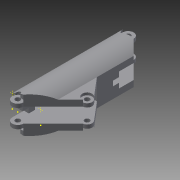
# Autodesk Inventor part: Finger_Lower_main_1
Saved by Autodesk Inventor 2015 (Build 190159000, 159)
## iProperties
Created: 2016-07-06
Part Number: Finger_Lower_main_1
Material: Generic
Document SubType Name: Modeling
Designer: Neelotpal Nag
Density: 1 g/cm^3
Appearance: Default
Author: Neelotpal Nag
Autodesk Inventor part; units mm, degrees
ref_plane "YZ Plane" through (0, 0, 0) normal (1, 0, 0) x (0, 1, 0)
ref_plane "XZ Plane" through (0, 0, 0) normal (0, 1, 0) x (-1, 0, 0)
sketch "Sketch1" plane through (0, 0, 0) normal (0, 0, 1) x (1, 0, 0)
  line L0 (0, 0) -> (0, 45)
  line L1 (0, 0) -> (14.1421, 14.1421)
  line L2 (0, 0) -> (20, 0) construction
  line L3 (14.1421, 14.1421) -> (0, 14.1421)
  circle A0 centre (0, 0) radius 1
  circle A1 centre (14.1421, 14.1421) radius 1
  circle A2 centre (0, 45) radius 1
  circle A3 centre (0, 0) radius 2.25
  circle A4 centre (0, 45) radius 2.25
  dimension "d0" = 45
  dimension "d1" = 20
  dimension "d2" = 45
  dimension "d3" = 2
  dimension "d4" = 2
  dimension "d5" = 2
  dimension "d6" = 4.5
  dimension "d10" = 4.5
  constraints: 8 coincident, 8 end point, 5 centre point, 1 equal length, 1 horizontal, 1 perpendicular, 1 point on line, 1 vertical
  measures "d0" distance of L0.start L0.end
  measures "d1" distance of L1.start L1.end
  measures "d2" angle of L2 L1
  measures "d3" diameter of A0
  measures "d4" diameter of A1
  measures "d5" diameter of A2
  measures "d6" diameter of A3
  measures "d10" diameter of A4
ref_plane "Work Plane1" through (0, 0, 3) normal (0, 0, 1) x (1, 0, 0)
sketch "Sketch2" plane through (0, 0, 3) normal (0, 0, 1) x (1, 0, 0)
  circle A0 centre (0, 0) radius 1 projected
  circle A1 centre (0, 0) radius 2.25 projected
  circle A2 centre (14.1421, 14.1421) radius 1 projected
  circle A3 centre (0, 45) radius 1 projected
  circle A4 centre (0, 45) radius 2.25 projected
  line L0 (0, 0) -> (0, 45) projected
extrude "Extrusion1" add sketch "Sketch2" along normal blind 1.5 contours A1
sketch "Sketch3" plane through (0, 0, 3) normal (0, 0, 1) x (1, 0, 0)
  point P0 (0, 0)
extrude "Extrusion2" add sketch "Sketch2" along normal blind 1.5 contours A4
sketch "Sketch4" plane through (0, 0, 3) normal (0, 0, 1) x (1, 0, 0)
  circle A0 centre (0, 0) radius 2.25 projected
  line L0 (-2.25, 0) -> (-2.25, 45)
  circle A1 centre (0, 45) radius 2.25 projected
  line L1 (2.25, 45) -> (9.3211, 37.9289)
  line L2 (2.25, 45) -> (12.25, 45) construction
  line L3 (9.3211, 37.9289) -> (9.3211, 22.9289)
  dimension "d13" = 10
  dimension "d14" = 45
  dimension "d15" = 15
  constraints: 8 end point, 2 point on circle, 1 equal length, 1 horizontal, 1 horizontal alignment, 1 parallel, 1 tangent, 1 vertical, 1 other
  measures "d13" distance of L1.start L1.end
  measures "d14" angle of L1 L2
  measures "d15" distance of L1.end L3.end
sketch "Sketch5" plane through (0, 0, 3) normal (0, 0, 1) x (1, 0, 0)
  circle A0 centre (14.1421, 14.1421) radius 1 projected
  circle A1 centre (14.1421, 14.1421) radius 2
  point P0 (0, 0)
  dimension "d16" = 4
  constraints: 1 centre point, 1 coincident
  measures "d16" diameter of A1
extrude "Extrusion3" add sketch "Sketch5" along normal blind 1.5
sketch "Sketch6" plane through (0, 0, 3) normal (0, 0, 1) x (1, 0, 0)
  circle A0 centre (0, 45) radius 2.25 projected
  line L0 (2.25, 45) -> (9.3211, 37.9289)
  line L1 (2.25, 45) -> (12.25, 45) construction
  line L2 (9.3211, 37.9289) -> (9.3211, 22.9289)
  line L3 (9.3211, 22.9289) -> (15.6683, 15.4347)
  circle A1 centre (14.1421, 14.1421) radius 2 projected
  line L4 (-2.25, 45) -> (-2.25, 0)
  circle A2 centre (0, 0) radius 2.25 projected
  circle A3 centre (14.1421, 14.1421) radius 2 projected
  circle A4 centre (14.1421, 14.1421) radius 1 projected
  line L5 (2.25, 0) -> (14.4102, 12.1602)
  line L6 (2.25, 0) -> (19.4471, 0) construction
  arc A5 (-2.25, 45) -> (2.25, 45) centre (0, 45) ccw
  line L7 (2.25, 45) -> (9.3211, 37.9289)
  line L8 (9.3211, 22.9289) -> (9.3211, 37.9289)
  line L9 (9.3211, 22.9289) -> (15.6683, 15.4347)
  line L10 (14.4102, 12.1602) -> (2.25, 0)
  circle A6 centre (14.1421, 14.1421) radius 2
  circle A7 centre (0, 0) radius 2.25
  line L11 (-2.25, 0) -> (-2.25, 45)
  circle A8 centre (0, 45) radius 2.25
  arc A9 (-2.25, 45) -> (2.25, 45) centre (0, 45) ccw
  arc A10 (15.6683, 15.4347) -> (14.4102, 12.1602) centre (14.1421, 14.1421) ccw
  arc A11 (2.25, 0) -> (-2.25, 0) centre (0, 0) ccw
  dimension "d19" = 10
  dimension "d20" = 45
  dimension "d21" = 15
  dimension "d22" = 45
  constraints: 24 end point, 12 point on circle, 7 centre point, 7 tangent, 6 concentric, 3 coincident, 3 collinear, 2 equal length, 2 horizontal, 1 vertical, 7 other
  measures "d19" distance of L0.start L0.end
  measures "d20" angle of L0 L1
  measures "d21" distance of L0.end L2.end
  measures "d22" angle of L6 L5
extrude "Extrusion4" add sketch "Sketch6" along normal blind 2.5 contours L0 L2 L3 A1 L5 A2 L4 A0
mirror "Mirror1" about plane through (0, 0, 0) normal (0, 0, 1) of "Extrusion4"
mirror "Mirror2" about plane through (0, 0, 0) normal (0, 0, 1) of "Extrusion2", "Extrusion3", "Extrusion1"
sketch "Sketch7" plane through (-2.25, 0, -5.5) normal (-1, 0, 0) x (0, 0, 1)
  point P0 (5.5, 0)
sketch "Sketch9" plane through (9.3211, 22.9289, -3) normal (1, 0, 0) x (0, 0, -1)
  line L0 (-6, 13.0711) -> (0, 13.0711)
  line L1 (0, 13.0711) -> (0, 0)
  line L2 (0, 0) -> (-6, 0)
  line L3 (-6, 0) -> (-6, 13.0711)
  point P0 (-3, -22.9289)
  constraints: 8 end point, 2 parallel, 1 horizontal, 1 perpendicular
extrude "Extrusion6" add sketch "Sketch9" against normal blind 2
sketch "Sketch12" plane through (9.3211, 22.9289, 5.5) normal (1, 0, 0) x (0, 0, -1)
  line L0 (8.5, 13.0711) -> (2.5, 13.0711) projected
  line L1 (6.5, 7.0711) -> (6.5, -16.9289) projected
  line L2 (4.5, 13.0711) -> (6.5, 13.0711)
  line L3 (6.5, 13.0711) -> (6.5, 6.5711)
  line L4 (6.5, 6.5711) -> (4.5, 6.5711)
  line L5 (4.5, 6.5711) -> (4.5, 13.0711)
  line L6 (8.5, 22.0711) -> (8.5, -22.9289) projected
  line L7 (2.5, 13.0711) -> (8.5, 13.0711)
  line L8 (8.5, 13.0711) -> (8.5, 9.0711)
  line L9 (8.5, 9.0711) -> (2.5, 9.0711)
  line L10 (2.5, 9.0711) -> (2.5, 13.0711)
  point P0 (5.5, -22.9289)
  point P1 (5.5, 13.0711)
  dimension "d50" = 6.5
  dimension "d61" = 4
  constraints: 16 end point, 4 parallel, 3 point on line, 2 horizontal, 2 perpendicular, 1 midpoint
  measures "d50" distance of L2.end L3.end
  measures "d61" distance of L7.end L8.end
extrude "Extrusion9" cut sketch "Sketch12" against normal blind 3 contours L3 L9 L5 L0 | L3 L1 L4 L5 L9
sketch "Sketch14" plane through (-2.25, 0, 3) normal (-1, 0, 0) x (0, 0, 1)
  line L0 (0, 45) -> (0, 0) projected
  line L1 (-6, 45) -> (-6, 0) projected
  line L2 (-6, 2.25) -> (0, 2.25)
  line L3 (-7.5, 0) -> (-7.5, 2.25) projected
  line L4 (-6, 2.25) -> (-6, 7.25)
  line L5 (-6, 7.25) -> (0, 7.25)
  line L6 (0, 0) -> (0, 12.1602) projected
  line L7 (-6, 4.75) -> (0, 4.75)
  line L8 (-2, 2.25) -> (-4, 2.25)
  line L9 (-4, 2.25) -> (-4, 4.75)
  line L10 (-4, 4.75) -> (-2, 4.75)
  line L11 (-2, 4.75) -> (-2, 2.25)
  line L12 (-6, 7.25) -> (0, 7.25)
  line L13 (0, 7.25) -> (0, 4.75)
  line L14 (0, 4.75) -> (-6, 4.75)
  line L15 (-6, 4.75) -> (-6, 7.25)
  line L16 (-4, 4.75) -> (-2, 4.75)
  line L17 (-2, 4.75) -> (-2, 2.25)
  line L18 (-2, 2.25) -> (-4, 2.25)
  line L19 (-4, 2.25) -> (-4, 4.75)
  point P0 (-3, 0)
  point P1 (-3, 2.25)
  dimension "d53" = 5
  dimension "d54" = 2
  constraints: 32 end point, 7 point on line, 6 parallel, 6 perpendicular, 3 horizontal, 2 midpoint
  measures "d53" distance of L2.start L4.end
  measures "d54" distance of L9.end L10.end
extrude "Extrusion10" add sketch "Sketch14" against normal blind 2 contours L0 L7 L1 L5 | L11 L2 L9 L7
sketch "Sketch15" plane through (0, 0, -3) normal (0, 0, 1) x (1, 0, 0)
  arc A0 (-2.25, 45) -> (2.25, 45) centre (0, 45) ccw projected
  circle A1 centre (0, 45) radius 1 projected
  line L0 (-2.25, 45) -> (-2.25, 0) projected
  line L1 (-2.25, 42.75) -> (-2.25, 26.25)
  line L2 (0, 42.75) -> (0, 33.281)
  line L3 (0, 33.281) -> (0, 42.75)
  line L4 (0, 33.281) -> (-2.25, 26.25)
  line L5 (0, 42.75) -> (-2.25, 42.75)
  point P0 (0, 0)
  dimension "d57" = 16.5
  dimension "d58" = 9.469
  constraints: 10 end point, 2 point on line, 1 collinear, 1 horizontal, 1 point on circle, 1 vertical
  measures "d57" distance of L1.start L1.end
  measures "d58" distance of L2.start L2.end
extrude "Extrusion11" add sketch "Sketch15" along normal blind 6 contours A0 L5 L0 | L2 L4 L0 L5
sketch "Sketch16" plane through (-2.25, 0, 5.5) normal (-1, 0, 0) x (0, 0, 1)
  point P0 (-5.5, 0)
sketch "Sketch17" plane through (9.3211, 22.9289, 5.5) normal (1, 0, 0) x (0, 0, -1)
  point P0 (5.5, -22.9289)
sketch "Sketch18" plane through (9.3211, 22.9289, 5.5) normal (1, 0, 0) x (0, 0, -1)
  point P0 (5.5, -22.9289)
extrude "Extrusion12" cut sketch "Sketch12" against normal blind 4 contours L6 L9 L3 L0 | L3 L9 L5 L0 | L5 L9 L10 L0
sketch "Sketch19" plane through (0, 0, 0) normal (0, 1, 0) x (-1, 0, 0)
  point P0 (0, 0)
  point P1 (-9.3211, 5.5)
  point P2 (2.25, 5.5)
sketch "Sketch20" plane through (0, 0, 0) normal (0, 1, 0) x (-1, 0, 0)
  arc A0 (2.25, 5.5) -> (-9.3211, 5.5) centre (-3.5355, -2.6564) ccw
  line L0 (2.25, 5.5) -> (-9.3211, 5.5)
  line L1 (-15.6683, 5.5) -> (-9.3211, 5.5) projected
  line L2 (2.25, -3) -> (2.25, 3) projected
  line L3 (2.25, 0) -> (-9.3211, 0)
  line L4 (-9.3211, -1) -> (-9.3211, 1) projected
  arc A1 (-9.3211, -5.5) -> (2.25, -5.5) centre (-3.5355, 2.6564) ccw
  line L5 (2.25, -5.5) -> (-9.3211, -5.5)
  point P0 (0, 0)
  dimension "d64" = 10
  constraints: 6 end point, 4 point on circle, 3 symmetric about line, 2 centre point, 2 midpoint, 1 collinear, 1 other
  measures "d64" radius of A0
extrude "Extrusion13" add sketch "Sketch20" along normal blind 42.5
sketch "Sketch21" plane through (4.75, 42.5, -5.5) normal (0, 0, 1) x (1, 0, 0)
  line L0 (4.5711, -4.5711) -> (0, 0)
  line L1 (4.5711, -4.5711) -> (0, 0) projected
  line L2 (0, 0) -> (4.5711, 0)
  line L3 (4.5711, -4.5711) -> (4.5711, 0) projected
  line L4 (4.5711, 0) -> (4.5711, -4.5711)
  point P0 (-4.75, -42.5)
  constraints: 6 end point, 2 perpendicular, 1 collinear
extrude "Extrusion14" cut sketch "Sketch21" along normal mid plane 42.5
sketch "Sketch22" plane through (2.25, 0, -5.5) normal (0, 0, 1) x (1, 0, 0)
  line L0 (7.0711, 0) -> (7.0711, 7.0711)
  line L1 (0, 0) -> (7.0711, 7.0711) projected
  line L2 (0, 0) -> (7.0711, 0) projected
  line L3 (7.0711, 7.0711) -> (0, 0)
  line L4 (7.0711, 0) -> (7.0711, 7.0711)
  line L5 (7.0711, 0) -> (7.0711, 7.0711) projected
  point P0 (-2.25, 0)
  constraints: 6 end point, 2 collinear, 1 vertical
extrude "Extrusion15" cut sketch "Sketch22" along normal mid plane 42.5
extrude "Extrusion16" cut sketch "Sketch1" along normal mid plane 42.5 contours L1 A0 L0 | L0 A0 L1
ref_plane "Work Plane2" through (0, 0, 0) normal (0, 0, 1) x (1, 0, 0)
body "Solid1"
